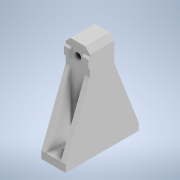
# Autodesk Inventor part: Soporte
Saved by Autodesk Inventor 2022 (Build 260153000, 153)
## iProperties
Created: 2021-04-28
Part Number: Soporte
Material: PET Plastic
Document SubType Name: Modeling
Designer: juanp
Density: 1.541 g/cm^3
Appearance: Polycarbonate - Clear
Author: juanp
Autodesk Inventor part; units mm, degrees
ref_plane "YZ Plane" through (0, 0, 0) normal (1, 0, 0) x (0, 1, 0)
ref_plane "XZ Plane" through (0, 0, 0) normal (0, 1, 0) x (-1, 0, 0)
ref_plane "XY Plane" through (0, 0, 0) normal (0, 0, 1) x (1, 0, 0)
sketch "Sketch5" plane through (0, 0, 0) normal (0, 1, 0) x (-1, 0, 0)
  line L0 (0, 0) -> (20, 0)
  line L1 (20, 0) -> (20, -20)
  line L2 (20, -20) -> (0, -20)
  line L3 (0, -20) -> (0, 0)
  dimension "d30" = 20
  dimension "d31" = 20
  constraints: 8 end point, 2 parallel, 1 horizontal, 1 perpendicular
  measures "d30" distance of L1.end L2.end
  measures "d31" distance of L0.end L1.end
extrude "Extrusion8" add sketch "Sketch5" along normal blind 76.2
sketch "Sketch6" plane through (-20, 0, 0) normal (0, 0, 1) x (1, 0, 0)
  line L0 (20, 76.2) -> (0, 76.2) projected
  line L1 (10, 76.2) -> (10, 66.2) construction
  circle A0 centre (10, 66.2) radius 2.65
  point P0 (20, 0)
  dimension "d34" = 10
  dimension "d35" = 5.3
  constraints: 2 end point, 1 centre point, 1 coincident, 1 midpoint, 1 vertical
  measures "d34" distance of L1.start L1.end
  measures "d35" diameter of A0
extrude "Extrusion9" cut sketch "Sketch6" against normal through all
sketch "Sketch7" plane through (-20, 0, 0) normal (0, 0, 1) x (1, 0, 0)
  line L0 (5, 66.2) -> (15, 66.2) construction
  circle A0 centre (10, 66.2) radius 2.65 projected
  line L1 (0, 70.575) -> (5, 70.575)
  line L2 (5, 70.575) -> (5, 61.825)
  line L3 (5, 61.825) -> (0, 61.825)
  line L4 (0, 61.825) -> (0, 70.575)
  line L5 (15, 70.575) -> (20, 70.575)
  line L6 (20, 70.575) -> (20, 61.825)
  line L7 (20, 61.825) -> (15, 61.825)
  line L8 (15, 61.825) -> (15, 70.575)
  line L9 (0, 0) -> (0, 76.2) projected
  point P0 (20, 0)
  dimension "d38" = 10
  dimension "d39" = 8.75
  constraints: 18 end point, 4 parallel, 3 horizontal, 3 midpoint, 2 equal length, 2 perpendicular, 1 coincident, 1 collinear
  measures "d38" distance of L0.end L0.start
  measures "d39" distance between parallel lines of L5 L7
extrude "Extrusion10" add sketch "Sketch7" along normal blind 1.35 contours L1 L2 L3 L4 | L5 L6 L7 L8
chamfer "Chamfer3" distance 1.35 angle 45 4 edges at (-2.5, 70.575, 1.35) (-2.5, 61.825, 1.35) (-17.5, 61.825, 1.35) (-17.5, 70.575, 1.35)
sketch "Sketch8" plane through (0, 0, 0) normal (0, -1, 0) x (1, 0, 0)
  line L0 (-20, -40) -> (0, -40)
  line L1 (0, -40) -> (0, 20)
  line L2 (0, 20) -> (-20, 20)
  line L3 (-20, 20) -> (-20, -40)
  line L4 (-20, -20) -> (-20, 0) projected
  line L5 (0, 0) -> (0, -20) projected
  line L6 (0, -20) -> (-20, -20) projected
  line L7 (-20, 0) -> (0, 0) projected
  line L8 (0, -40) -> (-20, -20) construction
  line L9 (-20, 0) -> (0, 20) construction
  circle A0 centre (-10, -30) radius 2.65
  circle A1 centre (-10, 10) radius 2.65
  point P0 (-20, -10)
  dimension "d45" = 60
  dimension "d46" = 5.3
  constraints: 12 end point, 4 midpoint, 2 centre point, 2 collinear, 2 parallel, 1 equal radius, 1 horizontal, 1 perpendicular
  measures "d45" distance of L2.end L0.start
  measures "d46" diameter of A1
extrude "Extrusion11" add sketch "Sketch8" against normal blind 4 contours L3 L6 L1 L0 | L3 L2 L1 L7
sketch "Sketch9" plane through (-20, 76.2, 0) normal (0, 0, 1) x (1, 0, 0)
  line L0 (20, -72.2) -> (0, -72.2) projected
  line L1 (0, -72.2) -> (0, -20)
  line L2 (0, -20) -> (4, -20)
  line L3 (4, -20) -> (4, -72.2)
  line L4 (16, -72.2) -> (16, -20)
  line L5 (16, -20) -> (20, -20)
  line L6 (20, -72.2) -> (20, -14.375) projected
  line L7 (20, -20) -> (20, -72.2)
  circle A0 centre (10, -10) radius 2.65 projected
  point P0 (20, -76.2)
  dimension "d49" = 10
  dimension "d50" = 4
  constraints: 12 end point, 4 point on line, 2 collinear, 2 perpendicular, 1 parallel, 1 vertical
  measures "d49" distance from line of L5 A0.centre
  measures "d50" distance of L4.end L5.end
ref_plane "Work Plane3" through (-20, 56.2, 0) normal (0, -0.35778, -0.9338059) x (1, 0, 0)
extrude "Extrusion12" add sketch "Sketch9" against normal up to surface contours L0 L4 L5 L6 | L0 L1 L2 L3 surface through (-20, 56.2, 0) normal (0, -0.35778, -0.9338059)
ref_plane "Work Plane4" through (-20, 76.2, -10) normal (0, 0, 1) x (1, 0, 0)
mirror "Mirror1" about plane through (-20, 76.2, -10) normal (0, 0, 1) of "Extrusion12"
chamfer "Chamfer4" distance 4 angle 45 2 edges at (-20, 76.2, -10) (0, 76.2, -10)
sketch "Sketch10" plane through (-4, 4, -20) normal (0, 0, -1) x (-1, 0, 0)
  circle A0 centre (6, 62.2) radius 2.65 projected
  circle A1 centre (6, 62.2) radius 4.25
  point P0 (-4, -4)
  dimension "d56" = 8.5
  constraints: 1 centre point, 1 coincident
  measures "d56" diameter of A1
extrude "Extrusion13" cut sketch "Sketch10" against normal blind 4
sketch "Sketch13" plane through (0, 0, 0) normal (0, -1, 0) x (1, 0, 0)
  circle A0 centre (-10, -30) radius 2.65 projected
  circle A1 centre (-10, 10) radius 2.65 projected
  line L0 (0, -40) -> (0, 20) projected
  line L1 (0, 20) -> (-20, 20) projected
  line L2 (-20, 20) -> (-20, -40) projected
  line L3 (-20, -40) -> (0, -40) projected
  point P0 (0, 0)
extrude "Extrusion15" add sketch "Sketch13" along normal blind 2 separate body
body "Solid2"
body "Solid4"
